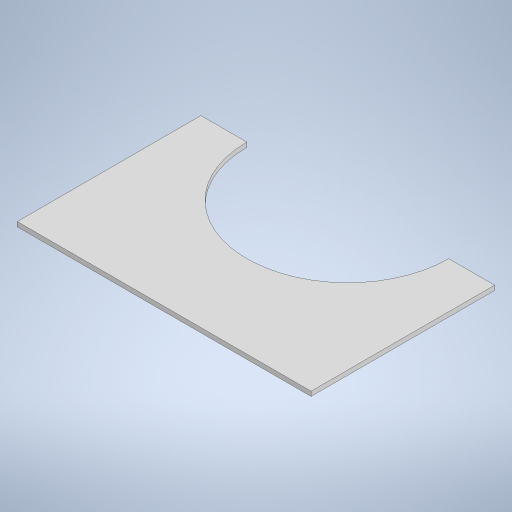
# Autodesk Inventor part: 2 Bottom Frame Base 2
Saved by Autodesk Inventor 2024 (Build 280153000, 153)
## iProperties
Created: 2024-04-17
Part Number: 2 Bottom Frame Base 2
Material: Generic
Document SubType Name: Modeling
Designer: Tommy Rohmann
Density: 1 g/cm^3
Appearance: Default
Author: Tommy Rohmann
Autodesk Inventor part; units mm, degrees
ref_plane "YZ Plane" through (0, 0, 0) normal (1, 0, 0) x (0, 1, 0)
ref_plane "XZ Plane" through (0, 0, 0) normal (0, 1, 0) x (-1, 0, 0)
ref_plane "XY Plane" through (0, 0, 0) normal (0, 0, 1) x (1, 0, 0)
sketch "Sketch1" plane through (0, 0, 0) normal (0, 1, 0) x (-1, 0, 0)
  line L0 (0, 0) -> (203.2, 0)
  line L1 (203.2, 0) -> (203.2, -254)
  line L2 (203.2, -254) -> (0, -254)
  line L3 (0, -254) -> (0, 0)
  line L4 (203.2, -127) -> (0, -127)
  line L5 (101.6, -254) -> (101.6, 0)
  circle A0 centre (101.6, -127) radius 69.85
  point P0 (171.45, -127)
  point P1 (31.75, -127)
  dimension "d0" = 203.2
  dimension "d1" = 254
  dimension "d2" = 139.7
  constraints: 12 end point, 5 midpoint, 2 parallel, 1 centre point, 1 horizontal, 1 perpendicular
  measures "d0" distance of L1.end L2.end
  measures "d1" distance of L0.end L1.end
  measures "d2" diameter of A0
extrude "Extrusion1" add sketch "Sketch1" along normal blind 3.175 contours L0 L5 A0 L4 L3 | L0 L1 L4 A0 L5
body "Solid1"
